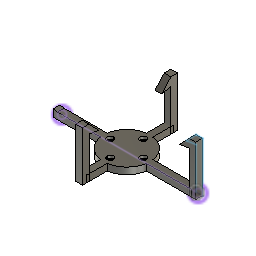
dome assembly (Autodesk Fusion 360 archive; units mm, degrees)
design "battery holder v5"
Autodesk Fusion 360 part; units mm, degrees
note: some values were not read from the file. Chosen so that the rebuilt part matches the saved one: which face or edge a step refers to; a side. Set by a fixed rule: which sketch regions a step uses.
sketch "Sketch1" plane through (0, 0, 0) normal (0, 0, 1) x (1, 0, 0) in component "battery bracket"
  circle A0 centre (0, 0) radius 17.5
  circle A1 centre (0.004, 12.5) radius 1.55
  circle A2 centre (-12.5, 0.004) radius 1.55
  circle A3 centre (-0.004, -12.5) radius 1.55
  circle A4 centre (12.5, -0.004) radius 1.55
  line L0 (51.5, -2.5) -> (-51.5, -2.5)
  line L1 (-51.5, -2.5) -> (-51.5, 2.5)
  line L2 (-51.5, 2.5) -> (51.5, 2.5)
  line L3 (51.5, 2.5) -> (51.5, -2.5)
  line L4 (51.5, -2.5) -> (-51.5, 2.5) construction
  line L5 (-51.5, -2.5) -> (51.5, 2.5) construction
  line L6 (2.5, 32.75) -> (-2.5, 32.75)
  line L7 (-2.5, 32.75) -> (-2.5, -32.75)
  line L8 (-2.5, -32.75) -> (2.5, -32.75)
  line L9 (2.5, -32.75) -> (2.5, 32.75)
  line L10 (2.5, 32.75) -> (-2.5, -32.75) construction
  line L11 (-2.5, 32.75) -> (2.5, -32.75) construction
  circle A5 centre (0.004, 12.5) radius 2.5
  circle A6 centre (12.5, -0.004) radius 2.5
  circle A7 centre (-0.004, -12.5) radius 2.5
  circle A8 centre (-12.5, 0.004) radius 2.5
  dimension "d5" = 35
  dimension "d7" = 3.1
  dimension "d9" = 360
  dimension "d10" = 12.5
  dimension "d13" = 103
  dimension "d15" = 5
  dimension "d18" = 5
  dimension "d19" = 65.5
  dimension "d61" = 5
  dimension "d62" = 5
  dimension "d63" = 5
  dimension "d64" = 5
  constraint coincident A0.centre origin
  constraint horizontal L0
  constraint perpendicular L0 L1
  constraint parallel L0 L2
  constraint parallel L1 L3
  constraint coincident L4 A0.centre
  constraint coincident L5 A0.centre
  constraint horizontal L6
  constraint perpendicular L6 L7
  constraint parallel L6 L8
  constraint parallel L7 L9
  constraint coincident L10 A0.centre
  constraint coincident L11 A0.centre
  constraint concentric A1 A5
  constraint concentric A4 A6
  constraint concentric A3 A7
  constraint concentric A2 A8
  measures "d5" diameter of A0
  measures "d7" diameter of A1
  measures "d10" vertical distance of A0.centre A1.centre
  measures "d13" distance of L0.start L0.end
  measures "d15" distance of L0 L2
  measures "d18" distance of L7.end L8.end
  measures "d19" distance of L6.end L7.end
  measures "d61" diameter of A5
  measures "d62" diameter of A6
  measures "d63" diameter of A7
  measures "d64" diameter of A8
extrude "Extrude1" add sketch "Sketch1" along normal blind 5 makes body 1 in component "battery bracket"
box "BoxPrimitive1" add length 65.5 width 103 height 25 placed x (0, -1, 0) y (1, 0, 0) z (0, 0, 1) at (-20, 0, 5) separate body makes body 2 in component "battery"
move_body "Move1" bodies 2 to x (1, 0, 0) y (0, 1, 0) z (0, 0, 1) at (-29.9229, 31.4243, 0.1248) in component "battery"
fillet "Fillet1" radius 2 4 faces at (-15.5895, 31.4243, 13.4581) (-15.5895, -34.0757, 13.4581) (-49.9229, -12.2424, 13.4581) (53.0771, -12.2424, 13.4581) on bodies 2 in component "battery"
fillet "Fillet1" radius 2 1 faces at (18.7438, 9.591, 5.1248) on bodies 2 in component "battery"
ref_plane "WorkPlane4" through (34.4103, 2.5, 2.5) normal (0, 1, 0) x (-1, 0, 0) in component "battery bracket"
sketch "Sketch3" plane through (0, 0, 0) normal (0, 0, 1) x (1, 0, 0) in component "battery bracket"
sketch "Sketch4" plane through (0, 2.5, 0) normal (0, 1, 0) x (1, 0, 0) in component "battery bracket"
  line L0 (54.9876, -37.6058) -> (49.9876, -37.6058)
  line L1 (49.9876, -31.1856) -> (49.9876, 0)
  line L2 (49.9876, 0) -> (54.9876, 0)
  line L3 (54.9876, 0) -> (54.9876, -37.6058)
  line L4 (-51.5, 0) -> (51.5, 0)
  line L5 (49.9876, -37.6058) -> (42.7828, -30)
  line L6 (42.7828, -30) -> (49.9876, -31.1856)
  dimension "d41" = 5
  dimension "d74" = 30
  constraint horizontal L0
  constraint vertical L1
  constraint horizontal L2
  constraint vertical L3
  constraint coincident L1.end L4
  constraint coincident L0.end L1
  measures "d41" distance of L1 L3
  measures "d74" distance of L4 L5.end
extrude "Extrude2" add sketch "Sketch4" against normal blind 5 separate body makes body 3 in component "battery bracket"
copy_body "CopyPasteBodies1" bodies 3 makes body 4
move_body "Move1'" bodies 4 to x (0.076138, 0.997097, 0) y (-0.997097, 0.076138, 0) z (0, 0, 1) at (38.2634, 47.4896, 0)
move_body "Move2" bodies 4 to x (1, 0, 0) y (0, 1, 0) z (0, 0, 1) at (-45.8694, -51.4609, 0)
move_body "Move3" bodies 4 to x (0.995524, 0.094509, 0) y (-0.094509, 0.995524, 0) z (0, 0, 1) at (8.0214, -14.2727, -0.1029)
copy_body "CutPasteBodies6" bodies 4 removing the originals makes body 5 in component "battery bracket"
mirror "Mirror1" about plane through (0, 0, 0) normal (0, 1, 0) of bodies 5 makes body 6 in component "battery bracket"
sketch "Sketch5" plane through (0, 2.5, 0) normal (0, 1, 0) x (1, 0, 0) in component "battery bracket"
  line L0 (-49.9743, 0) -> (-53.1211, 0)
  line L1 (-53.1211, 0) -> (-53.1211, -5.5925)
  line L2 (-53.1211, -5.5925) -> (-49.9743, -5)
  line L3 (-49.9743, -5) -> (-49.9743, 0)
  dimension "d51" = 5
  constraint horizontal L0
  constraint perpendicular L0 L1
  constraint vertical L3
  measures "d51" distance of L0.start L2.end
extrude "Extrude3" add sketch "Sketch5" against normal blind 5 bodies 1 in component "battery bracket"
move_body "Move4" bodies 3 to x (1, 0, 0) y (0, 1, 0) z (0, 0, 1) at (-0.2638, 0, 0) in component "battery bracket"
move_body "Move5" bodies 6 to x (1, 0, 0) y (0, 1, 0) z (0, 0, 1) at (0.0917, 0, 0) in component "battery bracket"
move_body "Move6" bodies 6 to x (1, 0, 0) y (0, 1, 0) z (0, 0, 1) at (0, 0, 0.0895) in component "battery bracket"
extrude "Extrude4" cut sketch "Sketch1" against normal blind 2 from surface at 5 contours L0 A6 | L9 A5 | L2 A8 | L7 A7 picked at (10.5378, 0.9434) picked at (2.163, 12.207) picked at (-14.4622, -0.9434) picked at (-2.163, -12.793) bodies 1 in component "battery bracket"
component "battery bracket" placed x (1, 0, 0) y (0, 1, 0) z (0, 0, 1) at (0, 0, 0)
component "battery" placed x (1, 0, 0) y (0, 1, 0) z (0, 0, 1) at (0, 0, 0)
equation "batt_outside_length = 103 mm"
equation "batt_outside_width = 65.5 mm"
equation "batt_outside_ht = 25 mm"
equation "pad_diam = 35 mm"
equation "d5 = pad_diam"
equation "m25_clearance_hole = 3.1 mm"
equation "d7 = m25_clearance_hole"
equation "tab_width = 5 mm"
equation "tab_thickness = 5 mm"
equation "d13 = batt_outside_length"
equation "d15 = tab_width"
equation "d16 = tab_thickness"
equation "d18 = tab_width"
equation "d19 = batt_outside_width"
equation "d23 = batt_outside_width"
equation "d24 = batt_outside_length"
equation "d25 = batt_outside_ht"
equation "clamp_width = 5 mm"
equation "post_width = 5 mm"
equation "post_thickness = 5 mm"
equation "clamp_extra = 8 mm"
equation "clamp_thickness = 5 mm"
equation "d41 = tab_thickness"
equation "d43 = -tab_width"
equation "d51 = tab_thickness"
equation "d52 = -tab_width"
equation "n25_head = 5 mm"
equation "d61 = n25_head"
equation "d62 = n25_head"
equation "d63 = n25_head"
equation "d64 = n25_head"
equation "d65 = tab_thickness"
equation "d74 = batt_outside_ht + tab_thickness"

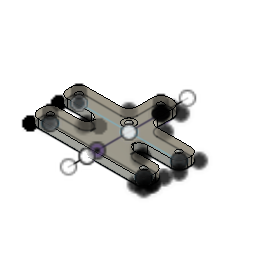
design "Lidar Holder V2"
Autodesk Fusion 360 part; units mm, degrees
sketch "Sketch1" plane through (0, 0, 0) normal (0, 0, 1) x (1, 0, 0) in component "Lidar Holder"
  line L0 (-8.2413, 25) -> (-8.2413, -25) construction
  line L1 (10.5767, 0) -> (88.2099, 0) construction
  line L2 (49.3933, 31.5) -> (49.3933, -31.5) construction
  line L3 (28.2492, 6) -> (28.2492, -6) construction
  circle A0 centre (49.3933, 31.5) radius 1.65
  line L4 (48.8209, 28.7) -> (51.5319, 29.6043)
  line L5 (51.5319, 29.6043) -> (52.1044, 32.4043)
  line L6 (52.1044, 32.4043) -> (49.9657, 34.3)
  line L7 (49.9657, 34.3) -> (47.2547, 33.3957)
  line L8 (47.2547, 33.3957) -> (46.6823, 30.5957)
  line L9 (46.6823, 30.5957) -> (48.8209, 28.7)
  line L10 (-10.9442, 24.0716) -> (-8.7888, 22.195)
  line L11 (-5.5384, 25.9284) -> (-7.6939, 27.805)
  line L12 (-7.6939, 27.805) -> (-10.3968, 26.8766)
  line L13 (-6.0859, 23.1234) -> (-5.5384, 25.9284)
  line L14 (-8.7888, 22.195) -> (-6.0859, 23.1234)
  circle A1 centre (-8.2413, 25) radius 1.65
  line L15 (-10.3968, 26.8766) -> (-10.9442, 24.0716)
  circle A2 centre (28.2492, 6) radius 1.65
  line L16 (25.5381, -6.9043) -> (27.6768, -8.8)
  line L17 (30.9602, 6.9043) -> (28.8216, 8.8)
  line L18 (27.6768, -8.8) -> (30.3878, -7.8957)
  line L19 (30.9602, -5.0957) -> (28.8216, -3.2)
  line L20 (26.1105, -4.1043) -> (25.5381, -6.9043)
  line L21 (27.6768, 3.2) -> (30.3878, 4.1043)
  line L22 (28.8216, 8.8) -> (26.1105, 7.8957)
  line L23 (25.5381, 5.0957) -> (27.6768, 3.2)
  line L24 (30.3878, -7.8957) -> (30.9602, -5.0957)
  circle A3 centre (28.2492, -6) radius 1.65
  line L25 (30.3878, 4.1043) -> (30.9602, 6.9043)
  line L26 (26.1105, 7.8957) -> (25.5381, 5.0957)
  line L27 (28.8216, -3.2) -> (26.1105, -4.1043)
  circle A4 centre (-8.2413, -25) radius 1.65
  line L28 (48.8209, -28.7) -> (51.5319, -29.6043)
  line L29 (51.5319, -29.6043) -> (52.1044, -32.4043)
  line L30 (-5.5384, -25.9284) -> (-7.6939, -27.805)
  line L31 (-10.3968, -26.8766) -> (-10.9442, -24.0716)
  line L32 (47.2547, -33.3957) -> (46.6823, -30.5957)
  line L33 (49.9657, -34.3) -> (47.2547, -33.3957)
  circle A5 centre (49.3933, -31.5) radius 1.65
  line L34 (52.1044, -32.4043) -> (49.9657, -34.3)
  line L35 (-8.7888, -22.195) -> (-6.0859, -23.1234)
  line L36 (-10.9442, -24.0716) -> (-8.7888, -22.195)
  line L37 (-6.0859, -23.1234) -> (-5.5384, -25.9284)
  line L38 (-7.6939, -27.805) -> (-10.3968, -26.8766)
  line L39 (46.6823, -30.5957) -> (48.8209, -28.7)
  line L40 (20.5675, -3.1744) -> (23.6233, -2.1184)
  line L41 (23.6233, -2.1184) -> (24.2367, 1.056)
  line L42 (18.7384, 2.1184) -> (18.125, -1.056)
  line L43 (24.2367, 1.056) -> (21.7943, 3.1744)
  circle A6 centre (21.1809, 0) radius 1.8
  line L44 (18.125, -1.056) -> (20.5675, -3.1744)
  line L45 (21.7943, 3.1744) -> (18.7384, 2.1184)
  line L46 (43.7384, 2.1184) -> (43.125, -1.056)
  circle A7 centre (46.1809, 0) radius 1.8
  line L47 (45.5675, -3.1744) -> (48.6233, -2.1184)
  line L48 (48.6233, -2.1184) -> (49.2367, 1.056)
  line L49 (43.125, -1.056) -> (45.5675, -3.1744)
  line L50 (46.7943, 3.1744) -> (43.7384, 2.1184)
  line L51 (49.2367, 1.056) -> (46.7943, 3.1744)
  point P0 (28.2492, 0)
  point P1 (49.3933, 31.5)
  point P2 (-8.2413, 25)
  point P3 (-8.2413, 25)
  point P4 (28.2492, -6)
  point P5 (28.2492, -6)
  point P6 (28.2492, 6)
  point P7 (28.2492, 6)
  point P8 (49.3933, -31.5)
  point P9 (-8.2413, -25)
  point P10 (-8.2413, -25)
  point P11 (49.3933, -31.5)
  point P12 (-8.2413, -25)
  point P13 (14, 0)
  point P14 (21.1809, 0)
  point P15 (46.1809, 0)
  point P16 (21.1809, 0)
  point P17 (21.1809, 0)
  point P18 (21.1809, 0)
  point P19 (46.1809, 0)
  point P20 (46.1809, 0)
  point P21 (46.1809, 0)
  point P22 (46.1809, 0)
  dimension "d1" = 50
  dimension "d2" = 63
  dimension "d3" = 58
  dimension "d5" = 58
  dimension "d6" = 12
  dimension "d7" = 3.3
  dimension "d8" = 2.475
  dimension "d11" = 3.3
  dimension "d12" = 2.475
  dimension "d13" = 3.3
  dimension "d14" = 2.475
  dimension "d15" = 3.3
  dimension "d16" = 2.475
  dimension "d43" = 25
  dimension "d45" = 3.6
  dimension "d46" = 2.8
  dimension "d48" = 3.6
  dimension "d49" = 2.8
  constraint vertical L0
  constraint perpendicular L0 L1
  constraint coincident origin L1
  constraint perpendicular L1 L2
  constraint midpoint L1 L2
  constraint perpendicular L1 L3
  constraint coincident L1 P0
  constraint coincident L3 P0
  constraint midpoint L3 P0
  constraint coincident P1 L2.start
  constraint coincident P3 P2
  constraint coincident P7 P6
  constraint coincident P5 P4
  constraint coincident P6 L3.start
  constraint coincident L3 P5
  constraint symmetric P3 L1 P12
  constraint symmetric L1 P1 P11
  constraint symmetric L1 A0 A5
  constraint symmetric L1 L4.start L28.start
  constraint symmetric L1 L4.end L28.end
  constraint symmetric L1 L5.end L29.end
  constraint symmetric L1 L6.end L33.start
  constraint symmetric L1 L7.end L32.start
  constraint symmetric L1 L8.end L32.end
  constraint symmetric L1 P3 P12
  constraint symmetric L1 L10.end L35.start
  constraint symmetric L1 L13.start L35.end
  constraint symmetric L1 L11.start L30.start
  constraint symmetric L1 L11.end L30.end
  constraint symmetric L1 L12.end L31.start
  constraint symmetric L1 L10.start L31.end
  constraint symmetric L1 A1 A4
  constraint coincident L1 P13
  constraint coincident L1 P18
  constraint coincident L1 P22
  constraint coincident P18 P17
  constraint coincident P22 P21
  measures "d1" distance of P3 P12
  measures "d2" distance of P1 P11
  measures "d3" distance of P3 L2.start
  measures "d5" distance of P12 P11
  measures "d6" distance of P6 P5
  measures "d7" diameter of A0
  measures "d8" distance of P1 L9
  measures "d11" diameter of A1
  measures "d12" distance of P3 L10
  measures "d13" diameter of A2
  measures "d14" distance of P7 L23
  measures "d15" diameter of A3
  measures "d16" distance of P5 L16
  measures "d43" distance of P18 P22
  measures "d45" diameter of A6
  measures "d46" distance of P18 L44
  measures "d48" diameter of A7
  measures "d49" distance of P22 L49
sketch "Sketch3" plane through (0, 0, 0) normal (0, 0, 1) x (1, 0, 0) in component "Lidar Holder"
  circle A0 centre (-8.3253, 24.9791) radius 7.5
  circle A1 centre (49.4758, 31.4678) radius 7.5
  line L0 (16.4935, 11.8388) -> (29.5378, 11.8388)
  line L1 (53.4093, 11.8388) -> (53.4093, 0.0068)
  line L2 (53.4093, 0.0068) -> (15.9047, 0.0068)
  line L3 (-12.4261, 18.6995) -> (2.6308, 8.1807)
  line L4 (12.8515, 13.4129) -> (-2.8624, 30.1179)
  line L5 (53.4093, 0.0068) -> (56.9268, 30.6115)
  line L6 (34.1277, 14.8556) -> (42.591, 34.4427)
  arc A2 (29.5378, 11.8388) -> (34.1277, 14.8556) centre (29.5378, 16.8388) ccw
  arc A3 (12.8515, 13.4129) -> (16.4935, 11.8388) centre (16.4935, 16.8388) ccw
  arc A4 (13.0412, 0.9079) -> (15.9047, 0.0068) centre (15.9047, 5.0068) ccw
  line L7 (10.5767, 0) -> (88.2099, 0)
  circle A5 centre (49.4758, -31.4678) radius 7.5
  line L8 (34.1277, -14.8556) -> (42.591, -34.4427)
  line L9 (53.4093, -0.0068) -> (56.9268, -30.6115)
  line L10 (53.4093, -0.0068) -> (15.9047, -0.0068)
  line L11 (16.4935, -11.8388) -> (29.5378, -11.8388)
  circle A6 centre (-8.3253, -24.9791) radius 7.5
  arc A7 (16.4935, -11.8388) -> (12.8515, -13.4129) centre (16.4935, -16.8388) ccw
  line L12 (12.8515, -13.4129) -> (-2.8624, -30.1179)
  line L13 (53.4093, -11.8388) -> (53.4093, -0.0068)
  line L14 (-16.0959, -21.3585) -> (2.6488, -8.2021)
  arc A8 (34.1277, -14.8556) -> (29.5378, -11.8388) centre (29.5378, -16.8388) ccw
  arc A9 (15.9047, -0.0068) -> (13.0412, -0.9079) centre (15.9047, -5.0068) ccw
  arc A10 (2.6488, -8.2021) -> (2.6308, 8.1807) centre (-3.0961, -0.017) ccw
  line L15 (-14.2071, -0.8825) -> (56.8712, 0.5267)
  dimension "d65" = 15
  dimension "d66" = 15
  dimension "d67" = 5
  dimension "d68" = 10
  constraint horizontal L0
  constraint vertical L1
  constraint horizontal L2
  constraint coincident A0 L4.end
  constraint tangent A0 L4
  constraint coincident A1 L5.end
  constraint tangent A1 L5
  constraint coincident L1.start L0
  constraint tangent L6 A2
  constraint tangent L0 A2
  constraint tangent L4 A3
  constraint tangent L0 A3
  constraint equal A2 A3
  constraint tangent L3 A4
  constraint tangent L2 A4
  constraint equal A2 A4
  constraint symmetric A0 L7 A6
  constraint symmetric A1 L7 A5
  constraint symmetric L1.start L7 L13.start
  constraint symmetric L1.end L7 L9.start
  constraint symmetric L4.end L7 L12.end
  constraint symmetric L5.end L7 L9.end
  constraint symmetric L6.end L7 L8.end
  constraint symmetric L6.start L7 L8.start
  constraint symmetric L0.end L7 L11.end
  constraint symmetric A2 L7 A8
  constraint symmetric L4.start L7 A7.end
  constraint symmetric L0.start L7 L11.start
  constraint symmetric A3 L7 A7
  constraint symmetric A4.start L7 A9.end
  constraint symmetric L2.end L7 L10.end
  constraint symmetric A4 L7 A9
  constraint coincident L3 A4.start
  constraint coincident A9.end L14
  constraint tangent L3 A10
  constraint tangent L14 A10
  constraint coincident A1 L6.end
  constraint tangent A1 L6
  constraint coincident A0 L3.start
  measures "d65" diameter of A0
  measures "d66" diameter of A1
  measures "d67" radius of A2
  measures "d68" radius of A10
extrude "Extrude4" add sketch "Sketch3" sketch "Sketch1" along normal blind 4 of sketch 2 contours A0 | L4 L5 L6 L7 L8 L9 | L10 L11 L12 L13 L14 L15 | A1 | A2 | L16 L18 L19 L20 L24 L27 | L17 L21 L22 L23 L25 L26 | A3 | A4 | L28 L29 L32 L33 L34 L39 | L30 L31 L35 L36 L37 L38 | A5 | L40 L41 L42 L43 L44 L45 | A6 | L46 L47 L48 L49 L50 L51 | A7 makes body 1 in component "Lidar Holder"
extrude "Extrude5" cut sketch "Sketch1" along normal blind 4 contours A0 | A1 | A2 | A3 | A4 | A5 | A6 | A7 bodies 1 in component "Lidar Holder"
extrude "Extrude6" cut sketch "Sketch1" along normal blind 2 contours L40 L41 L42 L43 L44 L45 | L46 L47 L48 L49 L50 L51 bodies 1 in component "Lidar Holder"
extrude "Extrude7" cut sketch "Sketch1" against normal blind 2 from surface at 4 contours L4 L5 L6 L7 L8 L9 | L10 L11 L12 L13 L14 L15 | L16 L18 L19 L20 L24 L27 | L17 L21 L22 L23 L25 L26 | L28 L29 L32 L33 L34 L39 | L30 L31 L35 L36 L37 L38 bodies 1 in component "Lidar Holder"
sketch "lidar base holes" plane through (0, 0, 0) normal (0, 0, 1) x (1, 0, 0) in component "Ldrobot"
  line L0 (-23.4, 0) -> (23.4, 0)
  line L1 (0, 0) -> (0, 31.92)
  dimension "d78" = 46.8
  dimension "d79" = 31.92
  constraint horizontal L0
  constraint midpoint L1.start L0
  constraint coincident L1.start origin
  constraint perpendicular L0 L1
  measures "d78" distance of L0.start L0.end
  measures "d79" distance of L1.start L1.end
sketch "base grid holes" plane through (0, 0, 0) normal (0, 0, 1) x (1, 0, 0) in component "Ldrobot"
  line L0 (-25, 15.9809) -> (25, 15.9809)
  line L1 (0, 0) -> (0, 31.92)
  point P0 (0, 15.9809)
  dimension "d80" = 50
  constraint horizontal L0
  constraint coincident L0 P0
  constraint midpoint L0 P0
  constraint coincident L1 P0
  measures "d80" distance of L0.start L0.end
sketch "base" plane through (0, 0, 0) normal (0, 0, 1) x (1, 0, 0) in component "Ldrobot"
  line L0 (0, 36.92) -> (-1, 36.92)
  line L1 (-5, 32.92) -> (-5, 24.9809)
  line L2 (-9, 20.9809) -> (-26, 20.9809)
  line L3 (-30, 16.9809) -> (-30, 14.9809)
  line L4 (-26, 10.9809) -> (-14, 10.9809)
  line L5 (-10, 6.9809) -> (-10, 9)
  line L6 (-14, 5) -> (-24.4, 5)
  line L7 (-28.4, 1) -> (-28.4, -1)
  line L8 (-24.4, -5) -> (0, -5)
  line L9 (-25, 15.9809) -> (25, 15.9809)
  line L10 (-23.4, 0) -> (23.4, 0)
  line L11 (0, 45.2028) -> (0, -14.2581)
  arc A0 (-1, 36.92) -> (-5, 32.92) centre (-1, 32.92) ccw
  arc A1 (-9, 20.9809) -> (-5, 24.9809) centre (-9, 24.9809) ccw
  arc A2 (-26, 20.9809) -> (-30, 16.9809) centre (-26, 16.9809) ccw
  arc A3 (-10, 6.9809) -> (-14, 10.9809) centre (-14, 6.9809) ccw
  arc A4 (-30, 14.9809) -> (-26, 10.9809) centre (-26, 14.9809) ccw
  arc A5 (-14, 5) -> (-10, 9) centre (-14, 9) ccw
  arc A6 (-24.4, 5) -> (-28.4, 1) centre (-24.4, 1) ccw
  arc A7 (-28.4, -1) -> (-24.4, -5) centre (-24.4, -1) ccw
  circle A8 centre (-23.4, 0) radius 1.5
  circle A9 centre (-23.4, 0) radius 3
  circle A10 centre (-25, 15.9809) radius 3
  circle A11 centre (-25, 15.9809) radius 1.5
  circle A12 centre (-23.4, 0) radius 3
  circle A13 centre (-23.4, 0) radius 1.5
  circle A14 centre (-25, 15.9809) radius 1.5
  circle A15 centre (-0.0195, 15.9809) radius 3
  circle A16 centre (-0.0195, 15.9809) radius 1.5
  circle A17 centre (0, 31.92) radius 3
  circle A18 centre (0, 31.92) radius 1.5
  circle A19 centre (25, 15.9809) radius 1.5
  line L12 (0, 36.92) -> (1, 36.92)
  line L13 (28.4, 1) -> (28.4, -1)
  circle A20 centre (23.4, 0) radius 1.5
  circle A21 centre (25, 15.9809) radius 1.5
  arc A22 (28.4, 1) -> (24.4, 5) centre (24.4, 1) ccw
  circle A23 centre (0, 31.92) radius 3
  line L14 (26, 10.9809) -> (14, 10.9809)
  arc A24 (14, 10.9809) -> (10, 6.9809) centre (14, 6.9809) ccw
  circle A25 centre (23.4, 0) radius 3
  arc A26 (26, 10.9809) -> (30, 14.9809) centre (26, 14.9809) ccw
  circle A27 centre (23.4, 0) radius 1.5
  circle A28 centre (0.0195, 15.9809) radius 1.5
  line L15 (5, 32.92) -> (5, 24.9809)
  line L16 (10, 6.9809) -> (10, 9)
  circle A29 centre (25, 15.9809) radius 3
  line L17 (9, 20.9809) -> (26, 20.9809)
  arc A30 (5, 32.92) -> (1, 36.92) centre (1, 32.92) ccw
  circle A31 centre (23.4, 0) radius 3
  line L18 (30, 16.9809) -> (30, 14.9809)
  arc A32 (30, 16.9809) -> (26, 20.9809) centre (26, 16.9809) ccw
  line L19 (14, 5) -> (24.4, 5)
  arc A33 (10, 9) -> (14, 5) centre (14, 9) ccw
  arc A34 (5, 24.9809) -> (9, 20.9809) centre (9, 24.9809) ccw
  circle A35 centre (0.0195, 15.9809) radius 3
  circle A36 centre (0, 31.92) radius 1.5
  arc A37 (24.4, -5) -> (28.4, -1) centre (24.4, -1) ccw
  line L20 (24.4, -5) -> (0, -5)
  point P0 (-5, 36.92)
  point P1 (-30, 20.9809)
  point P2 (-30, 10.9809)
  point P3 (-10, 10.9809)
  point P4 (-28.4, 5)
  point P5 (-28.4, -5)
  point P6 (-23.4, 0)
  point P7 (-25, 15.9809)
  point P8 (0, 31.92)
  point P9 (0, 31.92)
  point P10 (0, 31.92)
  point P11 (23.4, 0)
  point P12 (5, 36.92)
  point P13 (10, 10.9809)
  point P14 (24.4, -5)
  point P15 (25, 15.9809)
  point P16 (24.4, -1)
  point P17 (28.4, 5)
  point P18 (25, 15.9809)
  point P19 (30, 20.9809)
  point P20 (28.4, -5)
  point P21 (23.4, 0)
  point P22 (0, 31.92)
  point P23 (30, 10.9809)
  point P24 (0, -5)
  dimension "d81" = 5
  dimension "d82" = 5
  dimension "d84" = 5
  dimension "d86" = 5
  dimension "d88" = 5
  dimension "d89" = 5
  dimension "d90" = 20
  dimension "thickness" = 4
  dimension "d105" = 3
  dimension "d106" = 6
  dimension "d107" = 3
  dimension "d108" = 6
  dimension "d109" = 3
  dimension "d110" = 6
  dimension "d111" = 3
  dimension "d112" = 6
  dimension "d113" = 3
  dimension "d114" = 6
  dimension "d115" = 3
  dimension "d117" = 10
  dimension "d118" = 10
  constraint horizontal L2
  constraint perpendicular L2 L3
  constraint perpendicular L3 L4
  constraint perpendicular L4 L5
  constraint perpendicular L5 L6
  constraint perpendicular L6 L7
  constraint perpendicular L7 L8
  constraint perpendicular L1 L2
  constraint coincident origin L11
  constraint coincident L0.start L11
  constraint horizontal L0
  constraint vertical L11
  constraint coincident P0 L1
  constraint coincident P0 L0
  constraint tangent L1 A0
  constraint tangent L0 A0
  constraint tangent L1 A1
  constraint tangent L2 A1
  constraint equal A0 A1
  constraint coincident P1 L2
  constraint coincident P1 L3
  constraint tangent L2 A2
  constraint tangent L3 A2
  constraint equal A0 A2
  constraint coincident P3 L4
  constraint coincident P3 L5
  constraint tangent L4 A3
  constraint tangent L5 A3
  constraint equal A0 A3
  constraint coincident P2 L3
  constraint coincident P2 L4
  constraint tangent L3 A4
  constraint tangent L4 A4
  constraint equal A0 A4
  constraint tangent L5 A5
  constraint tangent L6 A5
  constraint equal A0 A5
  constraint coincident P4 L6
  constraint coincident P4 L7
  constraint tangent L6 A6
  constraint tangent L7 A6
  constraint equal A0 A6
  constraint coincident P5 L7
  constraint coincident P5 L8
  constraint tangent L7 A7
  constraint tangent L8 A7
  constraint equal A0 A7
  constraint concentric A12 A13
  constraint coincident P7 L9.start
  constraint coincident P22 P10
  constraint symmetric L0.start L11 L12.start
  constraint symmetric P0 L11 P12
  constraint symmetric P1 L11 P19
  constraint symmetric P2 L11 P23
  constraint symmetric P3 L11 P13
  constraint symmetric P4 L11 P17
  constraint symmetric P5 L11 P20
  constraint symmetric P24 L11 L8.end
  constraint symmetric P6 L11 P21
  constraint symmetric P7 L11 P18
  constraint symmetric P22 L11 P10
  constraint symmetric L11 L1.start L15.start
  constraint symmetric L11 L0.end L12.end
  constraint symmetric L11 A0 A30
  constraint symmetric L11 L1.end L15.end
  constraint symmetric L11 L2.start L17.start
  constraint symmetric L11 A1 A34
  constraint symmetric L11 L2.end L17.end
  constraint symmetric L11 L3.start L18.start
  constraint symmetric L11 A2 A32
  constraint symmetric L11 L4.end L14.end
  constraint symmetric L11 L5.start A24.end
  constraint symmetric L11 A3 A24
  constraint symmetric L11 L3.end A26.end
  constraint symmetric L11 L4.start L14.start
  constraint symmetric L11 A4 A26
  constraint symmetric L11 L5.end L16.end
  constraint symmetric L11 L6.start L19.start
  constraint symmetric L11 A5 A33
  constraint symmetric L11 L6.end A22.end
  constraint symmetric L11 L7.start L13.start
  constraint symmetric L11 A6 A22
  constraint symmetric L11 L7.end L13.end
  constraint symmetric L11 L8.start P14
  constraint symmetric L11 A7.centre P16
  constraint symmetric L11 A8 A20
  constraint symmetric L11 A9 A25
  constraint symmetric L11 A10 A29
  constraint symmetric L11 A11 A19
  constraint symmetric L11 A12 A31
  constraint symmetric L11 A13 A27
  constraint symmetric L11 A14 A21
  constraint symmetric L11 A15 A35
  constraint symmetric L11 A16 A28
  constraint symmetric L11 A17 A23
  constraint symmetric L11 A18 A36
  constraint symmetric L11 P22 P10
  constraint symmetric L11 A7 A37
  measures "d81" distance of L7 P6
  measures "d82" distance of L3 P7
  measures "d84" distance of L4 L9
  measures "d86" distance of L8 L10
  measures "d88" vertical distance of L0.start P22
  measures "d89" distance of L0.start P0
  measures "d90" distance of P2 P3
  measures "thickness" radius of A0
  measures "d105" diameter of A8
  measures "d106" diameter of A9
  measures "d107" diameter of A11
  measures "d108" diameter of A10
  measures "d109" diameter of A13
  measures "d110" diameter of A12
  measures "d111" diameter of A14
  measures "d112" diameter of A15
  measures "d113" diameter of A16
  measures "d114" diameter of A17
  measures "d115" diameter of A18
  measures "d117" distance of L6 L8
  measures "d118" distance of L2 L4
extrude "Extrude11" add sketch "base" along normal blind 4 separate body contours L0 L1 L2 L3 L4 L6 L7 L8 L11 A0 A1 A2 A3 A4 A5 A6 A7 A15 A17 A23 | L11 A17 L12 L13 A22 A23 L14 A24 A26 L15 L17 A30 L18 A32 L19 A33 A34 A35 A37 L20 | L11 A17 A18 A23 A36 | L11 A17 A18 A23 A36 | L9 L11 A15 A28 | L9 L11 A16 A35 | L9 L11 A15 A28 | L9 L11 A16 A35 | A9 A12 | A10 | A25 A31 | A29 makes body 2 at (4.1005, -1.5405, 4)
extrude "Extrude12" cut sketch "base" along normal blind 2 contours L11 A17 A18 A23 A36 | L11 A17 A18 A23 A36 | A9 A12 | A25 A31 bodies 2
component "Lidar Holder" placed x (1, 0, 0) y (0, 1, 0) z (0, 0, 1) at (0, 0, 0)
component "Ldrobot" placed x (1, 0, 0) y (0, 1, 0) z (0, 0, 1) at (0, 0, 0)
equation "d7 = m25_hole_diam"
equation "d8 = m25_nut_diam / 2"
equation "m3_hole_diam = 3.6 mm"
equation "m3_nut_diam = 5.6 mm"
equation "d11 = m25_hole_diam"
equation "d12 = m25_nut_diam / 2"
equation "d13 = m25_hole_diam"
equation "d14 = m25_nut_diam / 2"
equation "d15 = m25_hole_diam"
equation "d16 = m25_nut_diam / 2"
equation "m3_nut_depth = 2 mm"
equation "plate_thickness = 4 mm"
equation "d45 = m3_hole_diam"
equation "d46 = m3_nut_diam / 2"
equation "d48 = m3_hole_diam"
equation "d49 = m3_nut_diam / 2"
equation "m25_hole_diam = 3.3 mm"
equation "m25_nut_diam = 4.95 mm"
equation "m25_nut_depth = 2 mm"
equation "d69 = plate_thickness"
equation "d71 = plate_thickness"
equation "d73 = m3_nut_depth"
equation "d75 = plate_thickness"
equation "d76 = -m25_nut_depth"
equation "d84 = tab_widtj / 2"
equation "d86 = tab_widtj / 2"
equation "d89 = tab_widtj / 2"
equation "tab_widtj = 10 mm"
equation "d117 = tab_widtj"
equation "d118 = tab_widtj"
equation "d119 = plate_thickness"

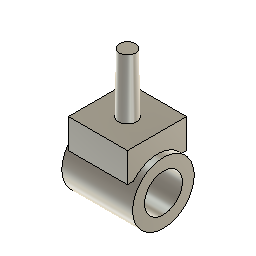
design "wire clip"
Autodesk Fusion 360 part; units mm, degrees
sketch "Sketch1" plane through (0, 0, 0) normal (0, 0, 1) x (1, 0, 0)
  circle A0 centre (0, 0) radius 3.25
  dimension "d1" = 6.5
  constraint coincident A0.centre origin
  measures "d1" diameter of A0
extrude "Extrude2" add sketch "Sketch1" along normal blind 10 draft -1 makes body 1
sketch "Sketch3" plane through (0, 0, 0) normal (0, 0, 1) x (1, 0, 0)
  line L0 (-5, -5) -> (5, -5)
  line L1 (5, -5) -> (5, 5)
  line L2 (5, 5) -> (-5, 5)
  line L3 (-5, 5) -> (-5, -5)
  line L4 (-5, -5) -> (5, 5) construction
  line L5 (5, -5) -> (-5, 5) construction
  dimension "d8" = 10
  dimension "d9" = 10
  constraint horizontal L0
  constraint perpendicular L0 L1
  constraint parallel L0 L2
  constraint parallel L1 L3
  constraint coincident L4 origin
  constraint coincident L5 origin
  measures "d8" distance of L1.end L2.end
  measures "d9" distance of L0.end L1.end
extrude "Extrude3" add sketch "Sketch3" against normal blind 5 bodies 1
sketch "Sketch4" plane through (0, 0, 0) normal (0, 1, 0) x (1, 0, 0)
  arc A0 (-0.732, 9.0567) -> (0.732, 9.0567) centre (0, 7.0886) ccw
  line L0 (0, 14.4265) -> (0, -9.1796) construction
  line L1 (-0.732, 9.0567) -> (0.732, 9.0567) construction
  dimension "d17" = 2.0998
  constraint vertical L0
  constraint coincident A0.centre L0
  constraint coincident origin L0
  constraint horizontal L1
  measures "d17" radius of A0
extrude "Extrude4" add sketch "Sketch4" along normal mid plane 8.494 thin wall 1 centred separate body open curves A0 makes body 2
ref_plane "WorkPlane2" through (0, 3, 0) normal (0, 1, 0) x (0, 0, 1)
ref_plane "WorkPlane3" through (0, -3, 0) normal (0, 1, 0) x (0, 0, 1)
sketch "Sketch5" plane through (0, -3, 0) normal (0, 1, 0) x (1, 0, 0)
  arc A0 (-4.9293, 3.6595) -> (-3.5699, 11.4787) centre (-0.767, 6.9637) ccw
sketch "Sketch6" plane through (0, 3, 0) normal (0, 1, 0) x (1, 0, 0)
  arc A0 (2.952, 10.8876) -> (4.3654, 5.2646) centre (-0.767, 6.9637) ccw
  point P0 (-0.767, 6.9637)
  constraint coincident P0 A0.centre
extrude "Extrude7" add sketch "Sketch6" along normal blind -1.5636 and the other way blind -1.377 thin wall 2 on the left open curves A0 bodies 1
extrude "Extrude5" add sketch "Sketch5" along normal blind 1.5271 and the other way blind 1.275 thin wall 2 on the left open curves A0 bodies 1
move_body "Move3" bodies 1 to x (1, 0, 0) y (0, 1, 0) z (0, 0, 1) at (0.6797, 0.6183, -0.8135)
move_body "Move4" bodies 1 to x (1, 0, 0) y (0, 1, 0) z (0, 0, 1) at (1.0478, 0, -1.0628)
move_body "Move5" bodies 1 to x (1, 0, 0) y (0, 1, 0) z (0, 0, 1) at (0, -0.6708, 0)
move_body "Move6" bodies 1 to x (1, 0, 0) y (0, 1, 0) z (0, 0, 1) at (-0.6735, 0, -0.5095)
copy_body "CopyPasteBodies1" bodies 1 makes body 3 in component "Printable"
move_body "Move1" bodies 3 to x (0.758843, 0, -0.651274) y (0, 1, 0) z (0.651274, 0, 0.758843) at (8.3155, 0, -6.6924) in component "Printable"
sketch "Sketch1 (2)" plane through (0, 0, 0) normal (0, 1, 0) x (1, 0, 0) in component "Printable"
  line L0 (3.95, -0.1916) -> (15.2555, -15.3312)
  line L1 (15.2555, -15.3312) -> (25.283, -0.1916)
  line L2 (25.283, -0.1916) -> (3.95, -0.1916)
  constraint horizontal L2
move_body "Move2" bodies 3 to x (1, 0, 0) y (0, 1, 0) z (0, 0, 1) at (0, 0, 19.9529) in component "Printable"
extrude "Extrude2'" add sketch "Sketch1 (2)" along normal mid plane 4 separate body makes body 4 in component "Printable"
move_body "Move3'" bodies 4 to x (1, 0, 0) y (0, 1, 0) z (0, 0, 1) at (2.3744, 0, 0) in component "Printable"
move_body "Move4'" bodies 3 to x (0.998428, 0, 0.056046) y (0, 1, 0) z (-0.056046, 0, 0.998428) at (0.6151, 0, -0.4069) in component "Printable"
box "BoxPrimitive1" add length 0.5 width 28.4805 height 10 placed x (0, 0, -1) y (-1, 0, 0) z (0, 1, 0) at (19.6199, 0, 0) separate body makes body 5 in component "Printable"
move_body "Move5'" bodies 5 to x (1, 0, 0) y (0, 1, 0) z (0, 0, 1) at (0, -4.562, 0) in component "Printable"
move_body "Move6'" bodies 5 to x (1, 0, 0) y (0, 1, 0) z (0, 0, 1) at (8.1898, 0, 0) in component "Printable"
sketch "Sketch5 (2)" plane through (0, 0, 0) normal (0, 1, 0) x (1, 0, 0) in component "Printable"
  line L0 (11.5323, -7.725) -> (8.4937, -3.7542)
  line L1 (8.4937, -3.7542) -> (11.5323, -7.725)
  line L2 (-0.6708, 0) -> (27.8097, 0)
  line L3 (27.8097, 0) -> (-0.6708, 0)
  line L4 (10.154, -5.9238) -> (11.8363, 0)
  constraint coincident L0 L4.start
  constraint coincident L3 L4.end
cylinder "CylinderPrimitive1" add diameter 0.5 height 3.7032 placed x (0.598334, 0, 0.801247) y (0, 1, 0) z (-0.801247, 0, 0.598334) at (15.0037, 0.0709, 11.8143) separate body makes body 6 in component "Printable"
cylinder "CylinderPrimitive2" add diameter 0.36 height 0.311 placed x (0.598334, 0, 0.801247) y (0, 1, 0) z (-0.801247, 0, 0.598334) at (9.8934, 0.0562, 4.971) bodies 4 in component "Printable"
move_body "Move7" bodies 1 to x (1, 0, 0) y (0, 1, 0) z (0, 0, 1) at (0.7865, 0, -0.217)
move_body "Move8" bodies 1 to x (1, 0, 0) y (0, 1, 0) z (0, 0, 1) at (-0.2441, 0, -0.4611)
sketch "Sketch1 (3)" plane through (0, 0, 0) normal (0, 0, 1) x (1, 0, 0) in component "biggerclosed"
  line L0 (5, -5) -> (-5, -5)
  line L1 (-5, -5) -> (-5, 5)
  line L2 (-5, 5) -> (5, 5)
  line L3 (5, 5) -> (5, -5)
  line L4 (5, -5) -> (-5, 5) construction
  line L5 (-5, -5) -> (5, 5) construction
  circle A0 centre (0, 0) radius 1.55
  dimension "d59" = 10
  dimension "d60" = 10
  dimension "d61" = 3.1
  constraint horizontal L0
  constraint perpendicular L0 L1
  constraint parallel L0 L2
  constraint parallel L1 L3
  constraint coincident L4 A0.centre
  constraint coincident L5 A0.centre
  constraint coincident A0.centre origin
  measures "d59" distance of L1.end L2.end
  measures "d60" distance of L0.end L1.end
  measures "d61" diameter of A0
extrude "Extrude1" add sketch "Sketch1 (3)" along normal blind 10 draft -1 separate body contours A0 makes body 7 in component "biggerclosed"
extrude "Extrude2''" add sketch "Sketch1 (3)" against normal blind 5 separate body contours L0 L1 L2 L3 | A0 makes body 8 in component "biggerclosed"
sketch "Sketch3 (2)" plane through (0, 0, 0) normal (1, 0, 0) x (0, 1, 0) in component "biggerclosed"
  circle A0 centre (0.0891, -8.2417) radius 3.2
  dimension "d66" = 6.4
  measures "d66" diameter of A0
extrude "Extrude3'" add sketch "Sketch3 (2)" along normal mid plane 12 thin wall 2 outside bodies 8 in component "biggerclosed"
component "Printable" placed x (1, 0, 0) y (0, 1, 0) z (0, 0, 1) at (0, 0, 0)
component "biggerclosed" placed x (1, 0, 0) y (0, 1, 0) z (0, 0, 1) at (0, 0, 0)
hidden bodies 2 4 5 6
equation "peg_diam = 3.1 mm"
equation "base_edge = 10 mm"
equation "base_height = 5 mm"
equation "peg_height = 10 mm"
equation "peg_taper = 1 deg"
equation "loop_extrude_distance = 6 mm"
equation "loop_extrude_wall = 2 mm"
equation "d59 = base_edge"
equation "d60 = base_edge"
equation "d61 = peg_diam"
equation "d62 = peg_height"
equation "d63 = -peg_taper"
equation "d64 = -base_height"
equation "d66 = loop_inside_diameter"
equation "d67 = loop_extrude_wall"
equation "d68 = loop_extrude_distance"
equation "loop_inside_diameter = 6.4 mm"

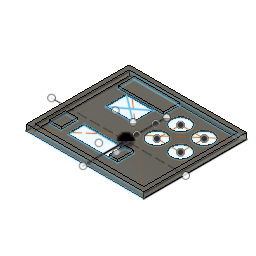
design "panel"
Autodesk Fusion 360 part; units mm, degrees
sketch "Sketch1" plane through (0, 0, 0) normal (0, 0, 1) x (1, 0, 0) in component "panel"
  line L0 (40, -27.916) -> (-40, -27.916)
  line L1 (-40, -27.916) -> (-40, 42.084)
  line L2 (-40, 42.084) -> (40, 42.084)
  line L3 (40, 42.084) -> (40, -27.916)
  line L4 (40, -27.916) -> (-40, 42.084) construction
  line L5 (-40, -27.916) -> (40, 42.084) construction
  line L6 (-8.572, 13.3986) -> (-27.072, 13.3986)
  line L7 (-27.072, 13.3986) -> (-27.072, 27.3986)
  line L8 (-27.072, 27.3986) -> (-8.572, 27.3986)
  line L9 (-8.572, 27.3986) -> (-8.572, 13.3986)
  line L10 (-8.572, 13.3986) -> (-27.072, 27.3986)
  line L11 (-37, 39.084) -> (37, 39.084)
  line L12 (37, 39.084) -> (37, -24.916)
  line L13 (37, -24.916) -> (-37, -24.916)
  line L14 (-37, -24.916) -> (-37, 39.084)
  line L15 (0, 27.7221) -> (0, -29.3166)
  line L16 (-50.7763, 0) -> (40.6939, 0) construction
  line L17 (-27.072, 13.3986) -> (-8.572, 27.3986)
  line L18 (4.1632, -15.7691) -> (-23.8368, -15.7691)
  line L19 (-23.8368, -15.7691) -> (-23.8368, -13.7732)
  line L20 (-23.8368, -4.7691) -> (4.1632, -4.7691)
  line L21 (4.1632, -4.7691) -> (4.1632, -15.7691)
  circle A0 centre (25.227, 28.1105) radius 7 construction
  circle A1 centre (9.0982, 28.1105) radius 7 construction
  circle A2 centre (9.0982, 11.9817) radius 7 construction
  circle A3 centre (25.227, 11.9817) radius 7 construction
  line L22 (9.0982, 28.1105) -> (25.227, 28.1105) construction
  line L23 (25.227, 28.1105) -> (25.227, 11.9817) construction
  line L24 (25.227, 11.9817) -> (9.0982, 11.9817) construction
  line L25 (9.0982, 11.9817) -> (9.0982, 28.1105) construction
  circle A4 centre (9.0982, 28.1105) radius 6.25
  circle A5 centre (25.227, 28.1105) radius 6.25
  circle A6 centre (9.0982, 11.9817) radius 6.25
  circle A7 centre (25.227, 11.9817) radius 6.25
  line L26 (10.0287, -15.7691) -> (10.0287, -4.7691)
  line L27 (-36.5408, -4.7691) -> (-36.5408, -15.7691)
  line L28 (-2.4014, 39.0876) -> (-33.2973, 39.0876)
  line L29 (-33.2973, 39.0876) -> (-33.2973, 28.1211)
  line L30 (-2.4014, 28.1211) -> (-2.4014, 39.0876)
  line L31 (-27.072, 13.3986) -> (-8.574, 13.3986)
  line L32 (-23.8368, -13.7732) -> (-23.8368, -4.7691)
  line L33 (-28.5221, -4.7691) -> (-28.5221, -15.7691)
  line L34 (10.0287, -4.7691) -> (-23.8368, -4.7691)
  line L35 (-28.5221, -4.7691) -> (-36.5408, -4.7691)
  line L36 (-36.5408, -15.7691) -> (-28.5221, -15.7691)
  line L37 (-23.8368, -15.7691) -> (10.0287, -15.7691)
  line L38 (-33.2973, 28.1211) -> (-2.4014, 28.1211)
  point P0 (-21.5849, 14.2567)
  point P1 (3.2352, -9.265)
  point P2 (0, 20.292)
  point P3 (0, 7.3263)
  point P4 (0, -24.916)
  point P5 (3.2509, -10.004)
  point P6 (-8.1386, -10.3752)
  dimension "d8" = 80
  dimension "d9" = 70
  dimension "d10" = 18.5
  dimension "d11" = 14
  dimension "d26" = 3
  dimension "d27" = 3
  dimension "d28" = 3
  dimension "d41" = 28
  dimension "d42" = 11
  dimension "d51" = 14
  dimension "d52" = 14
  dimension "d53" = 14
  dimension "d54" = 14
  dimension "d55" = 12.5
  dimension "d56" = 12.5
  dimension "d57" = 12.5
  dimension "d58" = 12.5
  dimension "d90" = 3
  constraint horizontal L0
  constraint perpendicular L0 L1
  constraint parallel L0 L2
  constraint parallel L1 L3
  constraint horizontal L6
  constraint perpendicular L6 L7
  constraint parallel L6 L8
  constraint parallel L7 L9
  constraint horizontal L11
  constraint vertical L12
  constraint horizontal L13
  constraint vertical L14
  constraint perpendicular L0 L15
  constraint coincident origin L15
  constraint perpendicular L3 L16
  constraint coincident origin L16
  constraint coincident L15 P2
  constraint coincident L15 P3
  constraint coincident L13 P4
  constraint coincident L15 P4
  constraint midpoint L13 P4
  constraint horizontal L18
  constraint perpendicular L18 L19
  constraint parallel L18 L20
  constraint parallel L19 L21
  constraint coincident A1.centre L22.start
  constraint perpendicular L22 L23
  constraint perpendicular L23 L24
  constraint coincident A2.centre L24.end
  constraint perpendicular L22 L25
  constraint coincident A0.centre L22.end
  constraint coincident A3.centre L23.end
  constraint horizontal L22
  constraint equal L24 L25
  constraint horizontal L36
  constraint vertical L26
  constraint horizontal L34
  constraint vertical L27
  constraint horizontal L28
  constraint vertical L29
  constraint horizontal L31
  constraint collinear L20 L34
  constraint collinear L18 L36
  constraint coincident L5 L19.end
  constraint perpendicular L18 L32
  constraint coincident L33.start L34
  constraint perpendicular L33 L36
  constraint perpendicular L30 L38
  measures "d8" distance of L1.end L2.end
  measures "d9" distance of L0.end L1.end
  measures "d10" distance of L7.end L8.end
  measures "d11" distance of L6.start L8.end
  measures "d26" distance of L2 L11
  measures "d27" distance of L0 L13
  measures "d28" distance of L1 L14
  measures "d41" distance of L20.start L20.end
  measures "d42" distance of L18 L20
  measures "d51" diameter of A0
  measures "d52" diameter of A1
  measures "d53" diameter of A2
  measures "d54" diameter of A3
  measures "d55" diameter of A4
  measures "d56" diameter of A5
  measures "d57" diameter of A6
  measures "d58" diameter of A7
  measures "d90" distance of L3 L12
extrude "Extrude1" add sketch "Sketch1" along normal blind 4 contours L0 L1 L2 L3 | L11 L12 L13 L14 L29 L30 L38 | L11 L28 L29 L30 | L11 L29 L30 L38 | L21 L26 L34 L37 | A4 | A5 | A6 | A7 | L27 L33 L35 L36 makes body 1
extrude "Extrude2" cut sketch "Sketch1" against normal blind 3.6 from surface at 4 contours L11 L12 L13 L14 L29 L30 L38 | L11 L29 L30 L38 | L15 L18 L20 L21 L34 L37 | L15 L18 L19 L20 L32 L34 L37 | L21 L26 L34 L37 | A4 | A5 | A6 | A7 | L27 L33 L35 L36 bodies 1
extrude "Extrude3" cut sketch "Sketch1" along normal blind 4 contours A4 | A5 | A6 | A7 bodies 1
sketch "Sketch3" plane through (40, 0, 0) normal (1, 0, 0) x (0, 1, 0)
  line L0 (-27.916, 0) -> (42.084, 0)
  line L1 (42.084, 0) -> (42.084, 4)
  line L2 (42.084, 4) -> (-27.916, 4)
  line L3 (-27.916, 4) -> (-27.916, 0)
  line L4 (-27.916, 0) -> (-6.2533, 20.8138)
  constraint coincident L0.start L3.end
extrude "Extrude5" add sketch "Sketch3" along normal blind 6 from surface at -6 thin wall 6 on the right separate body open curves L4 makes body 2
sketch "Sketch5" plane through (0, -9.2433, 9.6203) normal (0, 0.692836, -0.721095) x (-1, 0, 0)
  line L0 (-34, -20.1301) -> (-34, 9.9113)
  line L1 (-34, 9.9113) -> (-40, 9.9113)
  line L2 (-40, 9.9113) -> (-40, -20.1301)
  line L3 (-40, -20.1301) -> (-34, -20.1301)
ref_plane "WorkPlane3" through (0, 7.084, 2) normal (-1, 0, 0) x (0, -1, 0)
mirror "Mirror4" about plane through (0, 7.084, 2) normal (-1, 0, 0) of bodies 2 makes body 3
sketch "Sketch6" plane through (0, 0, 0) normal (0, 0, 1) x (1, 0, 0)
  line L0 (-29.9666, -19.5821) -> (3.6875, -19.5821)
  line L1 (3.6875, -19.5821) -> (3.6875, 0)
  line L2 (3.6875, 0) -> (-29.9666, 0)
  line L3 (-29.9666, 0) -> (-29.9666, -19.5821)
  line L4 (-31.1534, 8.5619) -> (-2.5855, 8.5619)
  line L5 (-2.5855, 8.5619) -> (-2.5855, 30.3481)
  line L6 (-2.5855, 30.3481) -> (-31.1534, 30.3481)
  line L7 (-31.1534, 30.3481) -> (-31.1534, 8.5619)
  constraint horizontal L0
  constraint vertical L1
  constraint horizontal L2
  constraint vertical L3
  constraint horizontal L4
  constraint vertical L5
  constraint horizontal L6
  constraint vertical L7
extrude "Extrude15" add sketch "Sketch1" along normal blind 2 contours L11 L29 L30 L38 | L21 L26 L34 L37 | L27 L33 L35 L36 bodies 1
component "panel" placed x (1, 0, 0) y (0, 1, 0) z (0, 0, 1) at (0, 0, 0)
hidden bodies 2 3
equation "small_oled_width = 28 mm"
equation "small_oled_ht = 11 mm"
equation "large_oled_ht = 14 mm"
equation "large_oled_width = 18.5 mm"
equation "panel_ht = 70 mm"
equation "panel_width = 80 mm"
equation "panel_thickness = 4 mm"
equation "d8 = panel_width"
equation "d9 = panel_ht"
equation "d10 = large_oled_width"
equation "d11 = large_oled_ht"
equation "indent_spacing = 3 mm"
equation "d26 = indent_spacing"
equation "d27 = indent_spacing"
equation "d28 = indent_spacing"
equation "sm_left_mg = 10 mm"
equation "d41 = small_oled_width"
equation "d42 = small_oled_ht"
equation "d45 = panel_thickness"
equation "d47 = -panel_thickness + 0.4 mm"
equation "btn_hole_diam = 12.5 mm"
equation "btn_clearance_diam = 14 mm"
equation "d51 = btn_clearance_diam"
equation "d52 = btn_clearance_diam"
equation "d53 = btn_clearance_diam"
equation "d54 = btn_clearance_diam"
equation "d55 = btn_hole_diam"
equation "d56 = btn_hole_diam"
equation "d57 = btn_hole_diam"
equation "d58 = btn_hole_diam"
equation "d59 = panel_thickness"
equation "screw_base_dua = 10 mm"
equation "d90 = indent_spacing"
equation "d118 = panel_thickness"
